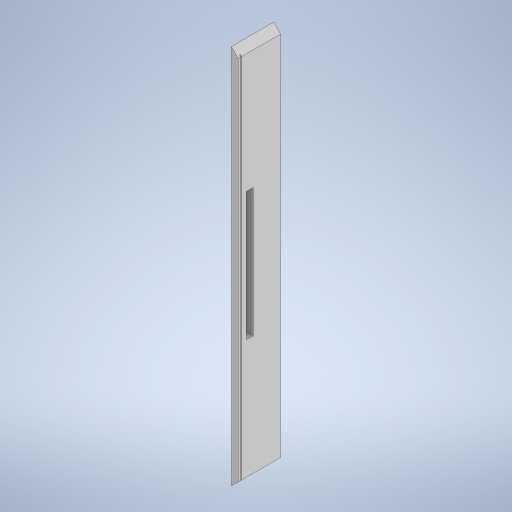
# Autodesk Inventor part: Frame Side(Short)
Saved by Autodesk Inventor 2024 (Build 280153000, 153)
## iProperties
Created: 2024-02-22
Part Number: Frame Side(Short)
Material: Generic
Document SubType Name: Modeling
Designer: flynf
Density: 1 g/cm^3
Appearance: Default
Author: flynf
Autodesk Inventor part; units mm, degrees
ref_plane "YZ Plane" through (0, 0, 0) normal (1, 0, 0) x (0, 1, 0)
ref_plane "XZ Plane" through (0, 0, 0) normal (0, 1, 0) x (-1, 0, 0)
ref_plane "XY Plane" through (0, 0, 0) normal (0, 0, 1) x (1, 0, 0)
sketch "Sketch1" plane through (0, 0, 0) normal (1, 0, 0) x (0, 1, 0)
  line L0 (0, 0) -> (1054.1, 0)
  line L1 (1054.1, 0) -> (1054.1, -22.225)
  line L2 (1054.1, -22.225) -> (0, -22.225)
  line L3 (0, -22.225) -> (0, 0)
  line L4 (349.25, -22.225) -> (349.25, -41.275)
  line L5 (349.25, -41.275) -> (704.85, -41.275)
  line L6 (704.85, -41.275) -> (704.85, -22.225)
  line L7 (349.25, -22.225) -> (0, -22.225)
  line L8 (0, -22.225) -> (0, -41.275)
  line L9 (0, -41.275) -> (349.25, -41.275)
  line L10 (349.25, -41.275) -> (349.25, -22.225)
  line L11 (704.85, -22.225) -> (1054.1, -22.225)
  line L12 (1054.1, -22.225) -> (1054.1, -41.275)
  line L13 (1054.1, -41.275) -> (704.85, -41.275)
  line L14 (704.85, -41.275) -> (704.85, -22.225)
  dimension "d0" = 1054.1
  dimension "d1" = 22.225
  dimension "d2" = 19.05
  dimension "d3" = 355.6
  dimension "d4" = 349.25
  constraints: 30 end point, 6 parallel, 5 perpendicular, 3 horizontal, 3 point on line, 1 vertical
  measures "d0" distance of L1.end L2.end
  measures "d1" distance of L0.end L1.end
  measures "d2" distance of L4.start L4.end
  measures "d3" distance of L4.end L5.end
  measures "d4" distance between parallel lines of L1 L6
extrude "Extrusion1" add sketch "Sketch1" along normal blind 19.05 contours L0 L1 L2 L3 | L2 L4 L9 L8 | L12 L13 L6 L2
sketch "Sketch2" plane through (19.05, 0, 0) normal (1, 0, 0) x (0, 0, -1)
  line L0 (41.275, 1054.1) -> (0, 1054.1) projected
  line L1 (0, 0) -> (41.275, 0) projected
  line L2 (6.35, 1054.1) -> (9.525, 1054.1)
  line L3 (9.525, 1054.1) -> (9.525, 0)
  line L4 (9.525, 0) -> (6.35, 0)
  line L5 (6.35, 0) -> (6.35, 1054.1)
  line L6 (0, 1054.1) -> (0, 0) projected
  point P0 (19.05, 1054.1)
  point P1 (19.05, 0)
  point P2 (6.35, 0)
  dimension "d7" = 3.175
  dimension "d8" = 6.35
  constraints: 8 end point, 2 parallel, 2 point on line, 1 horizontal, 1 perpendicular
  measures "d7" distance between parallel lines of L5 L3
  measures "d8" distance between parallel lines of L6 L5
extrude "Extrusion2" cut sketch "Sketch2" against normal blind 3.175 contours L3 L1 L5 L0
sketch "Sketch3" plane through (0, 0, 0) normal (0, 0, 1) x (1, 0, 0)
  line L0 (0, 0) -> (19.05, 19.05)
  line L1 (19.05, 1054.1) -> (19.05, 0) projected
  line L2 (0, 0) -> (26.9408, 0) construction
  line L3 (0, 1054.1) -> (19.05, 1035.05)
  line L4 (0, 1054.1) -> (26.9408, 1054.1) construction
  dimension "d11" = 45
  dimension "d12" = 45
  constraints: 8 end point, 2 equal length, 2 horizontal, 2 point on line
  measures "d11" angle of L2 L0
  measures "d12" angle of L3 L4
extrude "Extrusion3" cut sketch "Sketch3" against normal through all fills toward (9.5604, 9.4896) open curves L0
sketch "Sketch4" plane through (0, 0, 0) normal (0, 0, 1) x (1, 0, 0)
  line L0 (0, 349.25) -> (0, 704.85) projected
  line L1 (0, 1054.1) -> (19.05, 1035.05)
  line L2 (19.05, 1054.1) -> (19.05, 19.05) projected
  line L3 (0, 1054.1) -> (26.9408, 1054.1) construction
  point P0 (0, 0)
  dimension "d16" = 45
  constraints: 4 end point, 1 equal length, 1 horizontal, 1 point on line
  measures "d16" angle of L1 L3
extrude "Extrusion4" cut sketch "Sketch4" against normal through all fills toward (9.5604, 1044.6104) open curves L1
sketch "Sketch5" plane through (19.05, 704.85, -41.275) normal (0, 0, -1) x (-1, 0, 0)
  line L0 (19.05, 0) -> (19.05, 349.25) projected
  line L1 (19.05, 349.25) -> (0, 349.25)
  line L2 (0, 349.25) -> (0, -704.85)
  line L3 (0, -704.85) -> (19.05, -704.85)
  line L4 (19.05, -704.85) -> (19.05, 349.25)
  line L5 (19.05, -704.85) -> (0, -685.8) projected
  line L6 (19.05, -704.85) -> (0, -685.8)
  line L7 (0, 330.2) -> (19.05, 349.25) projected
  line L8 (19.05, 349.25) -> (0, 330.2)
  dimension "d20" = 19.05
  constraints: 12 end point, 3 equal length, 1 horizontal, 1 perpendicular, 1 point on line
  measures "d20" distance of L3.end L2.end
extrude "Extrusion5" add sketch "Sketch5" along normal blind 76.2 contours L4 L5 L2 L7 L0
body "Solid1"
